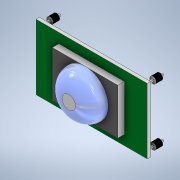
# Autodesk Inventor part: pir sensor
Saved by Autodesk Inventor 2021 (Build 250183000, 183)
## iProperties
Created: 2021-07-30
Part Number: pir sensor
Material: Generic
Document SubType Name: Modeling
Designer: user
Density: 1 g/cm^3
Appearance: Default
Author: user
Autodesk Inventor part; units mm, degrees
ref_plane "YZ Plane" through (0, 0, 0) normal (1, 0, 0) x (0, 1, 0)
ref_plane "XZ Plane" through (0, 0, 0) normal (0, 1, 0) x (-1, 0, 0)
ref_plane "XY Plane" through (0, 0, 0) normal (0, 0, 1) x (1, 0, 0)
sketch "Sketch1" plane through (0, 0, 0) normal (0, 0, 1) x (1, 0, 0)
  line L0 (17, -10) -> (-17, -10)
  line L1 (-17, -10) -> (-17, 10)
  line L2 (-17, 10) -> (17, 10)
  line L3 (17, 10) -> (17, -10)
  line L4 (17, -10) -> (-17, 10) construction
  line L5 (-17, -10) -> (17, 10) construction
  point P0 (0, 0)
  constraints: 12 end point, 2 midpoint, 2 parallel, 1 horizontal, 1 perpendicular
extrude "Extrusion1" add sketch "Sketch1" along normal blind 1
sketch "Sketch2" plane through (0, 0, 1) normal (0, 0, 1) x (1, 0, 0)
  line L0 (10, -7) -> (-10, -7)
  line L1 (-10, -7) -> (-10, 7)
  line L2 (-10, 7) -> (10, 7)
  line L3 (10, 7) -> (10, -7)
  line L4 (10, -7) -> (-10, 7) construction
  line L5 (-10, -7) -> (10, 7) construction
  point P0 (0, 0)
  constraints: 12 end point, 2 midpoint, 2 parallel, 1 horizontal, 1 perpendicular
extrude "Extrusion2" add sketch "Sketch2" along normal blind 2
sketch "Sketch3" plane through (0, 0, 3) normal (0, 0, 1) x (1, 0, 0)
  circle A0 centre (0, 0) radius 7.0711
  constraints: 1 centre point, 1 coincident
extrude "Extrusion3" add sketch "Sketch3" along normal blind 5
fillet "Fillet1" radius 5 1 edges at (-7.0711, 0, 8)
sketch "Sketch4" plane through (0, 0, 0) normal (0, 0, -1) x (-1, 0, 0)
  line L0 (16, -9) -> (15.5, -9)
  line L1 (15.5, -9) -> (15.5, -8.44)
  line L2 (15.5, -8.44) -> (16, -8.44)
  line L3 (16, -8.44) -> (16, -9)
  point P0 (0, 0)
  dimension "d7" = 0.5
  dimension "d8" = 0.56
  constraints: 8 end point, 2 parallel, 1 horizontal, 1 perpendicular
  measures "d7" distance of L1.end L2.end
  measures "d8" distance of L0.end L1.end
extrude "Extrusion4" add sketch "Sketch4" along normal blind 2
mirror "Mirror1" about plane through (0, 0, 0) normal (1, 0, 0) of "Extrusion4"
mirror "Mirror2" about plane through (0, 0, 0) normal (0, 1, 0) of "Extrusion4", "Mirror1"
sketch "Sketch5" plane through (0, 0, -2) normal (0, 0, -1) x (-1, 0, 0)
  circle A0 centre (15.75, -8.7479) radius 1
  point P0 (0, 0)
  dimension "d11" = 2
  constraints: 1 centre point
  measures "d11" diameter of A0
extrude "Extrusion5" add sketch "Sketch5" along normal blind 2
sketch "Sketch6" plane through (-15.75, -8.7479, -4) normal (0, 0, -1) x (-1, 0, 0)
  line L0 (-0.25, 0.25) -> (0.25, 0.25)
  line L1 (0.25, 0.25) -> (0.25, -0.25)
  line L2 (0.25, -0.25) -> (-0.25, -0.25)
  line L3 (-0.25, -0.25) -> (-0.25, 0.25)
  line L4 (-0.25, 0.25) -> (0.25, -0.25) construction
  line L5 (0.25, 0.25) -> (-0.25, -0.25) construction
  point P0 (-15.75, 8.7479)
  point P1 (0, 0)
  dimension "d14" = 0.5
  dimension "d15" = 0.5
  constraints: 12 end point, 2 midpoint, 2 parallel, 1 horizontal, 1 perpendicular
  measures "d14" distance of L1.end L2.end
  measures "d15" distance of L0.end L1.end
extrude "Extrusion6" add sketch "Sketch6" along normal blind 1
mirror "Mirror3" about plane through (0, 0, 0) normal (1, 0, 0) of "Extrusion6"
mirror "Mirror4" about plane through (0, 0, 0) normal (1, 0, 0) of "Extrusion6", "Extrusion5"
mirror "Mirror5" about plane through (0, 0, 0) normal (0, 1, 0) of "Extrusion5", "Extrusion6", "Mirror4"
sketch "Sketch7" plane through (0, 0, 1) normal (0, 0, 1) x (1, 0, 0)
  point P0 (0, 0)
ref_plane "Work Plane1" through (0, 0, 0) normal (0, 1, 0) x (-1, 0, 0)
body "Solid1"
